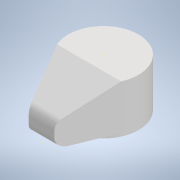
# Autodesk Inventor part: деталь2
Saved by Autodesk Inventor 2022 (Build 260153000, 153)
## iProperties
Created: 2021-04-16
Part Number: деталь2
Material: Типовые
Document SubType Name: Modeling
Designer: lbfas
Density: 1 g/cm^3
Appearance: По умолчанию
Author: lbfas
Autodesk Inventor part; units mm, degrees
ref_plane "YZ Plane" through (0, 0, 0) normal (1, 0, 0) x (0, 1, 0)
ref_plane "XZ Plane" through (0, 0, 0) normal (0, 1, 0) x (-1, 0, 0)
ref_plane "XY Plane" through (0, 0, 0) normal (0, 0, 1) x (1, 0, 0)
sketch "Эскиз1" plane through (0, 0, 0) normal (0, 1, 0) x (-1, 0, 0)
  arc A0 (-10.0374, 4.5) -> (10.0374, 4.5) centre (0, 0) ccw
  line L0 (0, 2) -> (-4.0311, 2)
  line L1 (0, 2) -> (4.0311, 2)
  arc A1 (-4.0311, 2) -> (4.0311, 2) centre (0, 0) ccw
  arc A2 (-4.0311, 2) -> (4.0311, 2) centre (0, 0) ccw
  line L2 (0, 4.5) -> (-10.0374, 4.5)
  line L3 (0, 4.5) -> (10.0374, 4.5)
  line L4 (-10.0374, 4.5) -> (-4.0311, 19.3918)
  line L5 (10.0374, 4.5) -> (4.0311, 19.3918)
  line L6 (-4.0311, 19.3918) -> (4.0311, 19.3918)
  dimension "d2" = 2
  constraints: 14 end point, 6 point on circle, 3 centre point, 2 coincident, 2 horizontal
  measures "d2" distance of A1.centre L0.start
extrude "Выдавливание1" add sketch "Эскиз1" along normal blind 14 contours L2 L3 A0 | L4 L6 L5 L3 L2 | L1 A1 L0
sketch "Эскиз2" plane through (0, 0, 0) normal (0, 1, 0) x (-1, 0, 0)
  arc A0 (-4.0311, 2) -> (4.0311, 2) centre (0, 0) ccw projected
  line L0 (4.0311, 2) -> (-4.0311, 2)
  constraints: 2 end point
sketch "Эскиз3" plane through (-4.0311, 0, 19.3918) normal (0, 0, 1) x (1, 0, 0)
  point P0 (4.0311, 0)
chamfer "Фаска1" distance 14.9 distance2 7 1 edges at (0, 14, 19.3918)
sketch "Эскиз4" plane through (0, 14, 0) normal (0, 1, 0) x (1, 0, 0)
  point P0 (0, 0)
fillet "Сопряжение1" radius 3 2 edges at (0, 7, 19.3918) (0, 0, 19.3918)
sketch "Эскиз5" plane through (0, 0, 0) normal (0, -1, 0) x (1, 0, 0)
  circle A0 centre (0, 0) radius 11
  arc A1 (-4.0311, 2) -> (4.0311, 2) centre (0, 0) ccw
  line L0 (4.0311, 2) -> (-4.0311, 2) projected
  line L1 (-4.0311, 2) -> (4.0311, 2)
  constraints: 2 centre point, 2 coincident, 2 end point, 2 point on circle, 1 collinear
extrude "Выдавливание2" add sketch "Эскиз5" along normal blind 1
sketch "Эскиз6" plane through (0, -1, 0) normal (0, -1, 0) x (1, 0, 0)
  point P0 (0, 0)
extrude "Выдавливание3" cut sketch "Эскиз2" along normal blind 9
